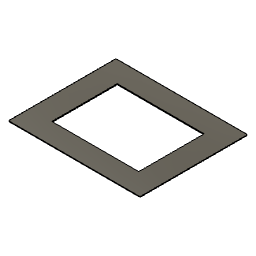
Window Mat (Autodesk Fusion 360 design; units mm, degrees)
Autodesk Fusion 360 part; units mm, degrees
sketch "Sketch1" plane through (0, 0, 0) normal (0, 0, 1) x (1, 0, 0)
  line L0 (0, 101) -> (134.5, 101)
  line L1 (134.5, 101) -> (134.5, 0)
  line L2 (134.5, 0) -> (205, 0)
  line L3 (205, 0) -> (205, 167.5)
  line L4 (205, 167.5) -> (0, 167.5)
  line L5 (0, 167.5) -> (0, 101)
  line L6 (-134.5, 101) -> (-134.5, 0)
  line L7 (-205, 0) -> (-205, 167.5)
  line L8 (-205, 167.5) -> (0, 167.5)
  line L9 (0, 101) -> (-134.5, 101)
  line L10 (0, 167.5) -> (0, 101)
  line L11 (-134.5, 0) -> (-205, 0)
  line L12 (134.5, -101) -> (134.5, 0)
  line L13 (205, -167.5) -> (0, -167.5)
  line L14 (0, -167.5) -> (0, -101)
  line L15 (0, -101) -> (-134.5, -101)
  line L16 (-134.5, 0) -> (-205, 0)
  line L17 (205, 0) -> (205, -167.5)
  line L18 (-205, 0) -> (-205, -167.5)
  line L19 (-205, -167.5) -> (0, -167.5)
  line L20 (-134.5, -101) -> (-134.5, 0)
  line L21 (0, -167.5) -> (0, -101)
  line L22 (0, -101) -> (134.5, -101)
  line L23 (134.5, 0) -> (205, 0)
  dimension "d26" = 101
  dimension "d27" = 134.5
  dimension "d28" = 101
  dimension "d29" = 70.5
  dimension "d30" = 167.5
  dimension "d31" = 205
  dimension "d32" = 66.5
  constraint perpendicular L0 L1
  constraint perpendicular L1 L2
  constraint perpendicular L2 L3
  constraint perpendicular L3 L4
  constraint perpendicular L4 L5
  constraint symmetric L0.start L5 L9.start
  constraint symmetric L0.end L5 L6.start
  constraint symmetric L1.end L5 L6.end
  constraint symmetric L2.end L5 L7.start
  constraint symmetric L3.end L5 L7.end
  constraint symmetric L4.end L5 L8.end
  constraint symmetric L0.start L2 L14.end
  constraint symmetric L0.end L2 L12.start
  constraint symmetric L1.end L2 L12.end
  constraint symmetric L3.start L2 L17.start
  constraint symmetric L2 L3.end L13.start
  constraint symmetric L2 L4.end L13.end
  constraint symmetric L2 L0.start L14.end
  constraint symmetric L2 L6.end L11.start
  constraint symmetric L2 L7.start L11.end
  constraint symmetric L2 L6.start L15.end
  constraint symmetric L2 L7.end L18.end
  measures "d26" distance of origin L0.start
  measures "d27" distance of L0.start L0.end
  measures "d28" distance of L0.end L1.end
  measures "d29" distance of L1.end L2.end
  measures "d30" distance of L2.end L3.end
  measures "d31" distance of L3.end L4.end
  measures "d32" distance of L4.end L0.start
extrude "Extrude4" add sketch "Sketch1" along normal blind 2 contours L0 L1 L2 L3 L4 L5 L10 L23 | L5 L6 L7 L8 L9 L10 L11 L16 | L2 L12 L13 L14 L17 L21 L22 L23 | L11 L14 L15 L16 L18 L19 L20 L21
chamfer "Chamfer2" distance 1 angle 45 4 edges at (0, 101, 2) (-134.5, 0, 2) (0, -101, 2) (134.5, 0, 2)
fillet "Fillet1" radius 2.5 4 edges at (205, -167.5, 1) (205, 167.5, 1) (-205, -167.5, 1) (-205, 167.5, 1)
